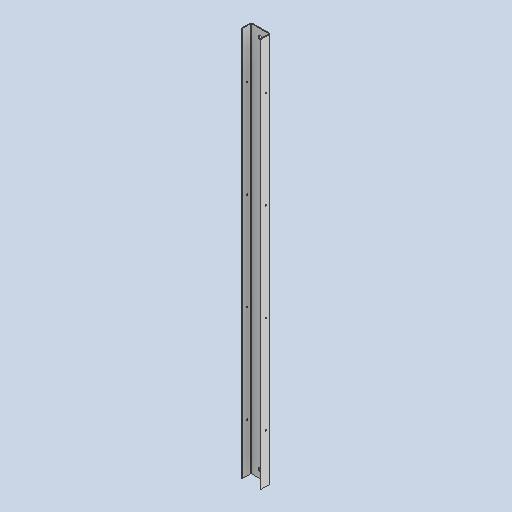
# Autodesk Inventor part: Beam_A1
Saved by Autodesk Inventor 2025.2 (Build 292293000, 293)
## iProperties
Created: 2025-03-13
Part Number: Beam_A1
Material: Generic
Document SubType Name: Sheet Metal
Designer: Andreas' PC
Density: 1 g/cm^3
Sheet Metal Rule: Default_mm
Appearance: Default
Author: Andreas' PC
Autodesk Inventor part; units mm, degrees
ref_plane "YZ Plane" through (0, 0, 0) normal (1, 0, 0) x (0, 1, 0)
ref_plane "XZ Plane" through (0, 0, 0) normal (0, 1, 0) x (-1, 0, 0)
ref_plane "XY Plane" through (0, 0, 0) normal (0, 0, 1) x (1, 0, 0)
sketch "Sketch1" plane through (0, 0, 0) normal (0, 0, 1) x (1, 0, 0)
  line L0 (0, 0) -> (50, 0)
  line L1 (50, 0) -> (50, 1000)
  line L2 (50, 1000) -> (0, 1000)
  line L3 (0, 1000) -> (0, 0)
  dimension "d0" = 50
  dimension "d1" = 1000
  measures "d0" distance of L2.end L1.end
  measures "d1" distance of L1.end L0.end
extrude "Plate1" add sketch "Sketch1" along normal blind 2
sketch "Sketch2" plane through (48, 1000, 0) normal (1, 0, 0) x (0, 1, 0)
  line L0 (-1000, 0) -> (0, 0)
  line L1 (0, 0) -> (0, 25)
  line L2 (0, 25) -> (-1000, 25)
  line L3 (-1000, 25) -> (-1000, 0)
  constraints: 6 end point, 1 horizontal, 1 perpendicular, 1 vertical
edge flange "Flange1" height 25 angle 90 thickness 2 bend radius 2 thickness toward (1, 0, 0) relief straight relief width 2 relief depth 1 edges at (50, 500, 2) wall of the first edge with corners at (48, 0, 0) (48, 1000, 0) (48, 1000, 25) (48, 0, 25)
bend "Bend1"
corner "Corner1"
sketch "Sketch3" plane through (2, 0, 0) normal (-1, 0, 0) x (0, -1, 0)
  line L0 (-1000, 0) -> (0, 0)
  line L1 (0, 0) -> (0, 25)
  line L2 (0, 25) -> (-1000, 25)
  line L3 (-1000, 25) -> (-1000, 0)
  constraints: 6 end point, 1 horizontal, 1 perpendicular, 1 vertical
edge flange "Flange2" height 25 angle 90 thickness 2 bend radius 2 thickness toward (-1, 0, 0) relief straight relief width 2 relief depth 1 edges at (0, 500, 2) wall of the first edge with corners at (2, 1000, 0) (2, 0, 0) (2, 0, 25) (2, 1000, 25)
bend "Bend2"
corner "Corner2"
sketch "Sketch4" plane through (0, 0, 25) normal (-1, 0, 0) x (0, 0, 1)
  circle A0 centre (-12.5, 125) radius 2
  line L0 (0, 0) -> (-21, 0) projected
  circle A1 centre (-12.5, 375) radius 2
  line L1 (-21, 1000) -> (-21, 0) projected
  circle A2 centre (-12.5, 625) radius 2
  circle A3 centre (-12.5, 875) radius 2
  line L2 (-21, 1000) -> (0, 1000) projected
  line L3 (-25, 1000) -> (-25, 0) projected
  dimension "d23" = 4
  dimension "d24" = 125
  dimension "d25" = 4
  dimension "d26" = 250
  dimension "d29" = 4
  dimension "d30" = 250
  dimension "d32" = 4
  dimension "d33" = 250
  dimension "d35" = 125
  dimension "d56" = 12.5
  dimension "d57" = 12.5
  dimension "d58" = 12.5
  dimension "d59" = 12.5
  constraints: 4 centre point
  measures "d23" diameter of A0
  measures "d24" distance from line of L0 A0.centre
  measures "d25" diameter of A1
  measures "d26" distance of A0.centre A1.centre
  measures "d29" diameter of A2
  measures "d30" distance of A1.centre A2.centre
  measures "d32" diameter of A3
  measures "d33" distance of A3.centre A2.centre
  measures "d35" distance from line of L2 A3.centre
  measures "d56" distance from line of L3 A0.centre
  measures "d57" distance from line of L3 A1.centre
  measures "d58" distance from line of L3 A2.centre
  measures "d59" distance from line of L3 A3.centre
hole "Hole1" at (0, 375, 12.5) at (0, 625, 12.5) at (0, 125, 12.5) at (0, 875, 12.5) direction (1, 0, 0) diameter 4 end through all
sketch "Sketch5" plane through (0, 0, 0) normal (0, 0, -1) x (-1, 0, 0)
  circle A0 centre (-25, 20) radius 5
  line L0 (-4, 0) -> (-46, 0) projected
  line L1 (0, 1000) -> (0, 0) projected
  circle A1 centre (-25, 980) radius 5
  line L2 (-46, 1000) -> (-4, 1000) projected
  dimension "d43" = 10
  dimension "d44" = 20
  dimension "d45" = 25
  dimension "d53" = 10
  dimension "d54" = 20
  dimension "d55" = 25
  constraints: 2 centre point
  measures "d43" diameter of A0
  measures "d44" distance from line of L0 A0.centre
  measures "d45" distance from line of L1 A0.centre
  measures "d53" diameter of A1
  measures "d54" distance from line of L2 A1.centre
  measures "d55" distance from line of L1 A1.centre
hole "Hole2" at (25, 20, 0) at (25, 980, 0) direction (0, 0, 1) diameter 10 end through all
equation "\"d0\" = A_height"
equation "\"d1\" = A_length"
equation "\"d23\" = rivet_diameter"
equation "\"d24\" = 0.5 * rivet_displacement"
equation "\"d25\" = rivet_diameter"
equation "\"d26\" = rivet_displacement"
equation "\"d29\" = rivet_diameter"
equation "\"d30\" = rivet_displacement"
equation "\"d32\" = rivet_diameter"
equation "\"d33\" = rivet_displacement"
equation "\"d56\" = 0.25 * A_width"
equation "\"d57\" = 0.25 * A_width"
equation "\"d58\" = 0.25 * A_width"
equation "\"d59\" = 0.25 * A_width"
equation "\"d36\" = rivet_diameter"
equation "\"d41\" = Thickness"
equation "\"d43\" = A_joint_diameter"
equation "\"d45\" = 0.5 * A_height"
equation "\"d53\" = A_joint_diameter"
equation "\"d55\" = 0.5 * A_height"
equation "\"d46\" = A_joint_diameter"
equation "\"d51\" = Thickness"
equation "\"d2\" = Thickness"
equation "\"d3\" = BendReliefWidth"
equation "\"d4\" = BendReliefDepth"
equation "\"d5\" = MinimumRemnant"
equation "\"d6\" = TransitionRadius"
equation "\"d7\" = 0.5 * A_width"
equation "\"d9\" = BendRadius"
equation "\"d10\" = CornerReliefSize"
equation "\"d11\" = GapSize"
equation "\"d12\" = JacobiRadiusSize"
equation "\"d13\" = BendReliefWidth"
equation "\"d14\" = BendReliefDepth"
equation "\"d15\" = MinimumRemnant"
equation "\"d16\" = TransitionRadius"
equation "\"d17\" = 0.5 * A_width"
equation "\"d19\" = BendRadius"
equation "\"d20\" = CornerReliefSize"
equation "\"d21\" = GapSize"
equation "\"d22\" = JacobiRadiusSize"
equation "\"Thickness\" = plate_thickness"
equation "\"BendRadius\" = Thickness"
equation "\"BendReliefWidth\" = Thickness"
equation "\"BendReliefDepth\" = 0.5 * Thickness"
equation "\"CornerReliefSize\" = 4 * Thickness"
equation "\"MinimumRemnant\" = 2 * Thickness"
equation "\"TransitionRadius\" = BendRadius"
equation "\"JacobiRadiusSize\" = BendRadius"
equation "\"GapSize\" = Thickness"
equation "\"A_length\" = 1000"
equation "\"l___________\" = 0"
equation "\"l__________\" = 0"
equation "\"l_________\" = 0"
equation "\"rivet_diameter\" = 4"
equation "\"rivet_displacement\" = 250"
equation "\"l________\" = 0"
equation "\"plate_thickness\" = 2"
equation "\"A_joint_diameter\" = 10"
equation "\"A_height\" = 50"
equation "\"A_joint_tolerance\" = 3"
equation "\"A_B_spacing\" = 2"
equation "\"L_Piston_Bottom\" = 21"
equation "\"L_Piston_Top\" = 25"
equation "\"A_width\" = 50"
body "Solid1"
